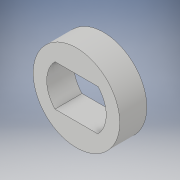
# Autodesk Inventor part: WheelCap
Saved by Autodesk Inventor 2018.3 (Build 223284000, 284)
## iProperties
Created: 2019-10-24
Part Number: WheelCap
Material: Generic
Document SubType Name: Modeling
Designer: j8qin
Density: 1 g/cm^3
Appearance: Default
Author: j8qin
Autodesk Inventor part; units mm, degrees
ref_plane "YZ Plane" through (0, 0, 0) normal (1, 0, 0) x (0, 1, 0)
ref_plane "XZ Plane" through (0, 0, 0) normal (0, 1, 0) x (-1, 0, 0)
ref_plane "XY Plane" through (0, 0, 0) normal (0, 0, 1) x (1, 0, 0)
sketch "Sketch1" plane through (0, 0, 0) normal (0, 0, 1) x (1, 0, 0)
  circle A0 centre (0, 0) radius 5.08
  circle A1 centre (0, 0) radius 0.88
  line L0 (-2.5268, -2.413) -> (2.523, -2.413)
  line L1 (2.523, 2.413) -> (-2.5268, 2.413)
  line L2 (-7.112, 0) -> (7.112, 0) projected
  arc A2 (2.523, -2.413) -> (2.523, 2.413) centre (-0.0019, 0) ccw
  arc A3 (-2.5268, 2.413) -> (-2.5268, -2.413) centre (-0.0019, 0) ccw
  dimension "d0" = 10.16
  dimension "d1" = 1.76
  dimension "d4" = 2.413
  dimension "d6" = 3.4925
  dimension "d7" = 3.4925
  dimension "d8" = 5.0498
  dimension "d9" = 2.413
  dimension "d10" = 2.413
  dimension "d12" = 4.826
  constraints: 4 centre point, 4 end point, 4 point on circle, 3 coincident, 1 horizontal, 1 parallel
  measures "d0" diameter of A0
  measures "d1" diameter of A1
  measures "d4" distance between parallel lines of L2 L1
  measures "d6" radius of A2
  measures "d7" radius of A3
  measures "d8" distance of L0.start L0.end
  measures "d9" distance from line of A3.centre L0
  measures "d10" distance from line of A2.centre L0
  measures "d12" distance between parallel lines of L1 L0
extrude "Extrusion3" add sketch "Sketch1" along normal mid plane 3.175 contours L2 A2 L1 A3 A0 | A0 L2 A3 L0 A2
body "Solid3"
